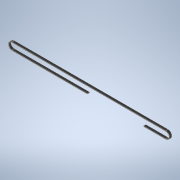
# Autodesk Inventor part: Riemen_T5
Saved by Autodesk Inventor 2022 (Build 260153000, 153)
## iProperties
Created: 2022-10-06
Part Number: Riemen_T5
Material: Gummi
Document SubType Name: Modeling
Designer: alexw
Mass: 23.1241 g
Surface Area: 192.513 cm^2
Volume: 24.8646 cm^3
Density: 0.93 g/cm^3
Appearance: Gummi - Schwarz
Author: alexw
Autodesk Inventor part; units mm, degrees
ref_plane "YZ Plane" through (0, 0, 0) normal (1, 0, 0) x (0, 1, 0)
ref_plane "XZ Plane" through (0, 0, 0) normal (0, 1, 0) x (-1, 0, 0)
ref_plane "XY Plane" through (0, 0, 0) normal (0, 0, 1) x (1, 0, 0)
sketch "Skizze1" plane through (0, 0, 0) normal (0, 0, 1) x (1, 0, 0)
  circle A0 centre (-380.0469, -116.0198) radius 3 construction
  circle A1 centre (-10.0469, -116.0198) radius 3.1 construction
  circle A2 centre (-380.0469, -116.0198) radius 9.05 construction
  circle A3 centre (-10.0469, -116.0198) radius 9.05 construction
  line L0 (-10.0469, -106.9698) -> (-380.0469, -106.9698)
  line L1 (-380.0469, -116.0198) -> (-380.0469, -106.9698) construction
  arc A4 (-380.0469, -106.9698) -> (-380.0469, -125.0698) centre (-380.0469, -116.0198) ccw
  line L2 (-380.0469, -125.0698) -> (-10.0469, -125.0698)
  arc A5 (-10.0469, -125.0698) -> (-10.0469, -106.9698) centre (-10.0469, -116.0198) ccw
  circle A6 centre (-380.0469, -116.0198) radius 7.65 construction
  circle A7 centre (-10.0469, -116.0198) radius 7.65 construction
  line L3 (-10.0469, -123.6698) -> (-380.0469, -123.6698)
  arc A8 (-380.0469, -108.3698) -> (-380.0469, -123.6698) centre (-380.0469, -116.0198) ccw
  line L4 (-380.0469, -108.3698) -> (-10.0469, -108.3698)
  arc A9 (-10.0469, -123.6698) -> (-10.0469, -108.3698) centre (-10.0469, -116.0198) ccw
  line L5 (-198.5469, -125.0698) -> (-198.5469, -123.6698)
  line L6 (-63.6869, -123.6698) -> (-63.6869, -125.0698)
  line L7 (-10.0469, -124.2698) -> (-380.0469, -124.2698) construction
  arc A10 (-380.0469, -107.7698) -> (-380.0469, -124.2698) centre (-380.0469, -116.0198) ccw construction
  line L8 (-380.0469, -107.7698) -> (-10.0469, -107.7698) construction
  arc A11 (-10.0469, -124.2698) -> (-10.0469, -107.7698) centre (-10.0469, -116.0198) ccw construction
  point P0 (0, 0)
  dimension "d0" = 370
  dimension "d3" = 370
  dimension "d8" = 53.64
  dimension "d9" = 181.5
  dimension "d11" = 181.5
  dimension "d12" = 370
  dimension "d13" = 53.64
  dimension "d14" = 8.25
  dimension "d15" = 8.25
  dimension "d16" = 15.3
  dimension "d17" = 15.3
  dimension "d18" = 0.8
  dimension "d19" = 1.4
  dimension "d20" = 18.1
  constraints: 20 point on circle, 18 end point, 12 centre point, 9 tangent, 6 point on line, 5 coincident, 3 perpendicular, 2 concentric, 1 vertical, 3 other
  measures "d0" distance of A1.centre A0.centre
  measures "d3" distance of A1.centre A0.centre
  measures "d8" distance from line of A1.centre L6
  measures "d9" distance from line of L5 A0.centre
  measures "d11" distance from line of L7.end L5
  measures "d12" distance of L8.end L8.start
  measures "d13" distance from line of L6 L7.start
  measures "d14" radius of A10
  measures "d15" radius of A11
  measures "d16" diameter of A6
  measures "d17" diameter of A7
  measures "d18" distance between parallel lines of L2 L7
  measures "d19" radial gap between concentric circles of A6 A2
  measures "d20" diameter of A2
extrude "Extrusion1" add sketch "Skizze1" along normal mid plane 6 contours A5 L2 L6 L3 A9 L4 A8 L5 A4 L0
equation "\"d8\" = Riemen_L_UpBottom"
equation "\"d9\" = Riemen_L_BottomUp"
equation "\"d17\" = d16"
equation "\"d2\" = d1"
equation "\"Riemen_L_UpBottom\" = 53.64"
equation "\"Bogenlaenge\" = 27.70885"
equation "\"Riemenlaenge\" = d12 + 2 * Bogenlaenge + d13 + d11"
equation "\"Riemen_L_BottomUp\" = 181.5"
equation "\"d1\" = 21.14"
